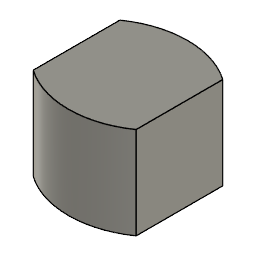
Motor (Autodesk Fusion 360 design; units mm, degrees)
part number: 2026-01-03-02-27-47-343
Autodesk Fusion 360 part; units mm, degrees
sketch "Motor base" plane through (0, 0, 0) normal (0, 0, 1) x (1, 0, 0)
  line L0 (0, 0) -> (0, -16)
  line L1 (0, -8) -> (-19, -8) construction
  line L2 (-9.5, -8) -> (-9.5, -19) construction
  line L3 (-19, 0) -> (-19, -16)
  arc A0 (-19, -16) -> (0, -16) centre (-9.5, -2.4583) ccw
  arc A1 (0, 0) -> (-19, 0) centre (-9.5, -13.5417) ccw
  dimension "d1" = 16
  dimension "d2" = 19
  dimension "d3" = 11
  constraint coincident L0.start A1.start
  constraint vertical L0
  constraint midpoint L0 L1.start
  constraint perpendicular L0 L1
  constraint midpoint L1 L2.start
  constraint perpendicular L1 L2
  constraint symmetric L0.start L2 L3.start
  constraint symmetric L0.end L2 L3.end
  constraint coincident L2.end A0
  constraint symmetric L0.end L1 L0.start
  constraint symmetric L1 L3.end L3.start
  constraint symmetric L1 A0 A1
  measures "d1" distance of L0.start L0.end
  measures "d2" distance of L1.start L1.end
  measures "d3" distance of L2.start L2.end
extrude "Motor height" add sketch "Motor base" along normal blind 17
equation "d1 = 22 mm - 6 mm"
named bodies: "Motor"
